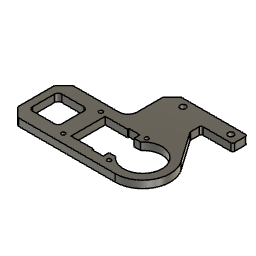
headcamera_plate_2R (Autodesk Fusion 360 design; units mm, degrees)
Autodesk Fusion 360 part; units mm, degrees
note: some values were not read from the file. Set by a fixed rule: which sketch regions a step uses; the direction of a hole.
sketch "スケッチ1" plane through (0, 0, 0) normal (0, 0, 1) x (1, 0, 0)
  line L0 (-53, -15) -> (0, -15)
  circle A0 centre (0, 0) radius 15
  line L1 (12.2873, 8.6036) -> (0.8064, 25)
  circle A1 centre (0, 0) radius 10.5
  line L2 (-33, 10.25) -> (-8, 10.25)
  line L3 (-8, 10.25) -> (-8, -10.25)
  line L4 (-8, -10.25) -> (-33, -10.25)
  line L5 (-33, -10.25) -> (-33, 10.25)
  line L6 (-13, 35) -> (13, 35)
  line L7 (-53, -15) -> (-58, -10)
  line L8 (-58, -10) -> (-58, 10)
  line L9 (-54, 8) -> (-38, 8)
  line L10 (-38, 8) -> (-38, -8)
  line L11 (-38, -8) -> (-54, -8)
  line L12 (-54, -8) -> (-54, 8)
  line L13 (-23, 15) -> (-53, 15)
  line L14 (-53, 15) -> (-58, 10)
  line L15 (-11.5, 10) -> (-11.5, -10)
  line L16 (-11.5, -10) -> (-17.5, -10)
  line L17 (-17.5, -10) -> (-17.5, -9.3)
  line L18 (-17.5, -9.3) -> (-29.7, -9.3)
  line L19 (-29.7, -9.3) -> (-29.7, 9.3)
  line L20 (-29.7, 9.3) -> (-17.5, 9.3)
  line L21 (-17.5, 9.3) -> (-17.5, 10)
  line L22 (-17.5, 10) -> (-11.5, 10)
  line L23 (-8, 6.8007) -> (-11.5, 6.8007)
  line L24 (-8, -6.8007) -> (-11.5, -6.8007)
  line L25 (0.8064, 25) -> (0.8064, 31)
  line L26 (0.8064, 31) -> (18, 31)
  line L27 (18, 31) -> (18, 39)
  line L28 (18, 39) -> (-18, 39)
  line L29 (-18, 39) -> (-23, 34)
  line L30 (-23, 34) -> (-23, 15)
  point P0 (-8, 0)
  point P1 (-11.5, 0)
  point P2 (-29.7, 0)
  point P3 (18, 35)
  dimension "d1" = 30
  dimension "d2" = 55
  dimension "d3" = 53
  dimension "d6" = 21
  dimension "d7" = 8
  dimension "d8" = 25
  dimension "d9" = 20.5
  dimension "d28" = 26
  dimension "d35" = 5
  dimension "d36" = 5
  dimension "d42" = 16
  dimension "d43" = 4
  dimension "d45" = 2
  dimension "d55" = 2
  dimension "d57" = 12.2
  dimension "d58" = 18.6
  dimension "d59" = 20
  dimension "d60" = 11.5
  dimension "d61" = 6
  dimension "d64" = 25
  dimension "d65" = 6
  dimension "d66" = 8
  dimension "d67" = 18
  dimension "d68" = 5
  dimension "d69" = 16
  dimension "d71" = 5
  dimension "d72" = 5
  dimension "d74" = 5
  dimension "d75" = 5
  dimension "d76" = 5
  constraint horizontal L0
  constraint coincident A0.centre A1.centre
  constraint coincident L0.end A0
  constraint tangent L0 A0
  constraint coincident A0 L1.start
  constraint tangent A0 L1
  constraint horizontal L2
  constraint vertical L3
  constraint horizontal L4
  constraint vertical L5
  constraint midpoint L3 P0
  constraint horizontal A0.centre P0
  constraint vertical L8
  constraint horizontal L9
  constraint vertical L10
  constraint horizontal L11
  constraint vertical L12
  constraint vertical L15
  constraint perpendicular L15 L16
  constraint perpendicular L16 L17
  constraint perpendicular L15 L18
  constraint perpendicular L18 L19
  constraint perpendicular L19 L20
  constraint perpendicular L18 L21
  constraint perpendicular L21 L22
  constraint coincident L15.start L22.end
  constraint midpoint L15 P1
  constraint horizontal A0.centre P1
  constraint midpoint L19 P2
  constraint horizontal P1 P2
  constraint coincident A1 L23.start
  constraint coincident L3 L23.start
  constraint coincident L15 L23.end
  constraint perpendicular L15 L23
  constraint coincident L3 L24.start
  constraint coincident A1 L24.start
  constraint coincident L15 L24.end
  constraint perpendicular L15 L24
  constraint vertical L25
  constraint perpendicular L25 L26
  constraint perpendicular L26 L27
  constraint perpendicular L27 L28
  constraint midpoint L27 P3
  constraint horizontal L6.end P3
  constraint horizontal L13
  constraint perpendicular L28 L30
  constraint coincident L13.start L30.end
  constraint horizontal L6
  measures "d1" diameter of A0
  measures "d2" angle of L0 L1
  measures "d3" distance of L0.start L0.end
  measures "d6" diameter of A1
  measures "d7" distance of A0.centre L3
  measures "d8" distance of L3.end L4.end
  measures "d9" distance of L2.start L4.end
  measures "d28" distance of L6.start L6.end
  measures "d35" horizontal distance of L0.start L7.end
  measures "d36" vertical distance of L0.start L7.end
  measures "d42" distance of L9.start L9.end
  measures "d43" distance of L8 L12
  measures "d45" distance of L7.end L11
  measures "d55" distance of L8.end L9
  measures "d57" distance of L19.end L20.end
  measures "d58" distance of L18.end L19.end
  measures "d59" distance of L16 L22
  measures "d60" distance of A0.centre L15
  measures "d61" distance of L21.end L15.start
  measures "d64" vertical distance of L1.end A0.centre
  measures "d65" distance of L1.end L25.end
  measures "d66" distance of L26.end L27.end
  measures "d67" distance of A0.centre L27
  measures "d68" distance of L6.end L27
  measures "d69" distance of L9.start L11.end
  measures "d71" vertical distance of L8.end L13.end
  measures "d72" horizontal distance of L8.end L13.end
  measures "d74" horizontal distance of L6.start L28.end
  measures "d75" horizontal distance of L28.end L29.end
  measures "d76" vertical distance of L28.end L29.end
extrude "押し出し1" add sketch "スケッチ1" along normal blind 4 contours L0 A0 L1 L2 L4 L5 L7 L8 L13 L14 L25 L26 L27 L28 L29 L30 | A0 A1 L2 L3 L4 | A0 L2 L4 L5 L15 L16 L17 L18 L19 L20 L21 L22 | A0 L3 L4 L15 L24 | A0 L2 L3 L15 L23
hole "穴1" at (-8, 10.25, 0) at (-8, -10.25, 0) at (-33, -10.25, 0) at (-33, 10.25, 0) direction (0, 0, 1) diameter 2.1 depth 10 tip angle 118
hole "穴3" at (-13, 35, 0) at (13, 35, 0) direction (0, 0, 1) diameter 3.2 depth 10 tip angle 118
fillet "フィレット3" radius 2 4 edges at (-54, 8, 2) (-54, -8, 2) (-38, -8, 2) (-38, 8, 2)
fillet "フィレット4" radius 1 10 edges at (-53, -15, 2) (-58, -10, 2) (-58, 10, 2) (-53, 15, 2) (-23, 34, 2) (-18, 39, 2) (18, 39, 2) (18, 31, 2) (0.8064, 25, 2) (0.8064, 31, 2)
fillet "フィレット5" radius 5 1 edges at (-23, 15, 2)
